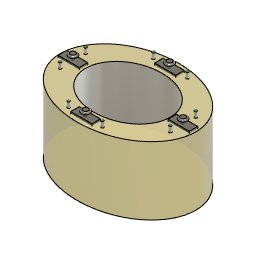
UCR Biohack 2021 - Neck Brace Outline v5 (Autodesk Fusion 360 design; units mm, degrees)
Autodesk Fusion 360 part; units mm, degrees
sketch "Sketch1" plane through (0, 0, 0) normal (0, 1, 0) x (1, 0, 0)
  ellipse E0 centre (0, 0) end of major axis (-50, 0) minor radius 40
  line L0 (50, 0) -> (-50, 0)
  line L1 (0, 40) -> (0, -40)
  ellipse E1 centre (0, 0) end of major axis (0.084, 59.9999) minor radius 80
  line L2 (-0.084, -59.9999) -> (0.084, 59.9999)
  line L3 (79.9999, -0.112) -> (-79.9999, 0.112)
  dimension "d1" = 100
  dimension "d2" = 80
  dimension "d3" = 60
  dimension "d4" = 80
  constraint horizontal L0
  constraint coincident E0 L0.start
  constraint coincident E0 L0.end
  constraint coincident E0 L1.start
  constraint coincident E0 L1.end
  constraint coincident E0.centre E1.centre
  constraint concentric E0 E1
  constraint coincident E1 L2.start
  constraint coincident E1 L2.end
  constraint coincident E1 L3.start
  constraint coincident E1 L3.end
  measures "d1" distance of E0
  measures "d3" distance of E1
extrude "Extrude1" add sketch "Sketch1" along normal blind 80 contours E0 E1 L2 L3 | E0 E1 L2 L3 | E0 E1 L2 L3 | E0 E1 L2 L3 makes body 1
sketch "Sketch4" plane through (0, 0, 0) normal (0, 1, 0) x (1, 0, 0)
  line L0 (-52.5, -5) -> (-77.5, -5)
  line L1 (-77.5, -5) -> (-77.5, 5)
  line L2 (-77.5, 5) -> (-52.5, 5)
  line L3 (-52.5, 5) -> (-52.5, -5)
  line L4 (-52.5, -5) -> (-77.5, 5) construction
  line L5 (-77.5, -5) -> (-52.5, 5) construction
  line L6 (77.5, -5.2811) -> (52.5, -5.2811)
  line L7 (52.5, -5.2811) -> (52.5, 4.7189)
  line L8 (52.5, 4.7189) -> (77.5, 4.7189)
  line L9 (77.5, 4.7189) -> (77.5, -5.2811)
  line L10 (77.5, -5.2811) -> (52.5, 4.7189) construction
  line L11 (52.5, -5.2811) -> (77.5, 4.7189) construction
  line L12 (12.3145, 44.0263) -> (-12.6855, 44.0263)
  line L13 (-12.6855, 44.0263) -> (-12.6855, 54.0263)
  line L14 (-12.6855, 54.0263) -> (12.3145, 54.0263)
  line L15 (12.3145, 54.0263) -> (12.3145, 44.0263)
  line L16 (12.3145, 44.0263) -> (-12.6855, 54.0263) construction
  line L17 (-12.6855, 44.0263) -> (12.3145, 54.0263) construction
  line L18 (12.5, -55) -> (-12.5, -55)
  line L19 (-12.5, -55) -> (-12.5, -45)
  line L20 (-12.5, -45) -> (12.5, -45)
  line L21 (12.5, -45) -> (12.5, -55)
  line L22 (12.5, -55) -> (-12.5, -45) construction
  line L23 (-12.5, -55) -> (12.5, -45) construction
  point P0 (-65, 0)
  point P1 (65, -0.2811)
  point P2 (-0.1855, 49.0263)
  point P3 (0, -50)
  constraint horizontal L0
  constraint perpendicular L0 L1
  constraint parallel L0 L2
  constraint parallel L1 L3
  constraint coincident L4 P0
  constraint coincident L5 P0
  constraint horizontal L6
  constraint perpendicular L6 L7
  constraint parallel L6 L8
  constraint parallel L7 L9
  constraint coincident L10 P1
  constraint coincident L11 P1
  constraint horizontal L12
  constraint perpendicular L12 L13
  constraint parallel L12 L14
  constraint parallel L13 L15
  constraint coincident L16 P2
  constraint coincident L17 P2
  constraint horizontal L18
  constraint perpendicular L18 L19
  constraint parallel L18 L20
  constraint parallel L19 L21
  constraint coincident L22 P3
  constraint coincident L23 P3
  constraint midpoint L22 P3
extrude "Extrude3" add sketch "Sketch4" along normal blind 82 separate body makes body 2 at (-4.3522, 27.3333, -54.0263) makes body 3 at (69.1667, 54.6667, 5.2811) makes body 4 at (-60.8333, 54.6667, 5) makes body 5 at (4.1667, 54.6667, 55)
sketch "Sketch5" plane through (0, 0, 0) normal (0, 1, 0) x (1, 0, 0)
  circle A0 centre (0, 49) radius 2.5
  circle A1 centre (0, -50) radius 2.5
  circle A2 centre (-65, 0) radius 2.5
  circle A3 centre (65, 0) radius 2.5
  dimension "d21" = 5
  dimension "d22" = 5
  dimension "d23" = 5
  dimension "d24" = 5
  measures "d21" diameter of A0
  measures "d22" diameter of A1
  measures "d23" diameter of A2
  measures "d24" diameter of A3
extrude "Extrude4" add sketch "Sketch5" along normal blind 86 separate body makes body 6 at (-2.3037, 57.3333, 50.9711) makes body 7 at (2.4969, 57.3333, -48.8754) makes body 8 at (-62.5031, 57.3333, 0.1246) makes body 9 at (67.4969, 57.3333, 0.1246)
sketch "Sketch7" plane through (0, 86, 0) normal (0, 1, 0) x (-1, 0, 0)
  circle A0 centre (-65, 0) radius 2.5
  circle A1 centre (-65, 0) radius 5
  circle A2 centre (0, -49) radius 5
  circle A3 centre (65, 0) radius 5
  circle A4 centre (0, 50) radius 5
  dimension "d31" = 10
  dimension "d32" = 10
  dimension "d33" = 10
  dimension "d34" = 10
  constraint concentric A0 A1
  measures "d31" diameter of A1
  measures "d32" diameter of A2
  measures "d33" diameter of A3
  measures "d34" diameter of A4
extrude "Extrude5" add sketch "Sketch7" along normal blind 2 contours A0 | A1 | A2 | A3 | A4 bodies 6 7 8 9
fillet "Fillet1" radius 2 4 edges at (4.6616, 88, 48.1919) (4.6616, 88, -50.8081) (-60.3384, 88, -1.8081) (69.6616, 88, -1.8081) on bodies 6 7 8 9
sketch "Sketch9" plane through (0, 80, 0) normal (0, 1, 0) x (-1, 0, 0)
  circle A0 centre (20, -50) radius 1.5
  circle A1 centre (-20, -50) radius 1.5
  circle A2 centre (65, -15) radius 1.5
  circle A3 centre (65, 15) radius 1.5
  circle A4 centre (20, 50) radius 1.5
  circle A5 centre (-20, 50) radius 1.5
  circle A6 centre (-65, 15) radius 1.5
  circle A7 centre (-65, -15) radius 1.5
  dimension "d43" = 3
  dimension "d44" = 3
  dimension "d45" = 3
  dimension "d46" = 3
  dimension "d47" = 3
  dimension "d48" = 3
  dimension "d49" = 3
  dimension "d50" = 3
  measures "d43" diameter of A0
  measures "d44" diameter of A1
  measures "d45" diameter of A2
  measures "d46" diameter of A3
  measures "d47" diameter of A4
  measures "d48" diameter of A5
  measures "d49" diameter of A6
  measures "d50" diameter of A7
extrude "Extrude6" add sketch "Sketch9" along normal blind 8 bodies 1
fillet "Fillet2" radius 1.5 8 edges at (-63.6015, 88, -15.5424) (-63.6015, 88, 14.4576) (-18.6015, 88, -50.5424) (21.3985, 88, -50.5424) (66.3985, 88, -15.5424) (66.3985, 88, 14.4576) (21.3985, 88, 49.4576) (-18.6015, 88, 49.4576) on bodies 1
